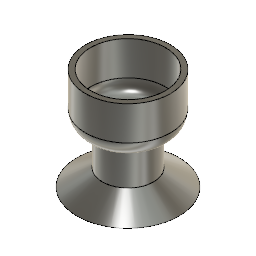
goblet v4 (Autodesk Fusion 360 design; units mm, degrees)
Autodesk Fusion 360 part; units mm, degrees
sketch "outline" plane through (0, 0, 0) normal (0, 1, 0) x (1, 0, 0)
  line L0 (25, -60) -> (25, -40)
  arc A0 (25, -40) -> (15, -30) centre (15, -40) ccw
  line L1 (15, -30) -> (15, -10)
  line L2 (15, -10) -> (30, 0)
  line L3 (30, 0) -> (10, 0)
  line L4 (22, -60) -> (22, -40)
  arc A1 (22, -40) -> (12, -33.6754) centre (15, -40) ccw
  line L5 (12, -33.6754) -> (12, -8.3944)
  line L6 (12, -8.3944) -> (20.0917, -3)
  line L7 (20.0917, -3) -> (10, -3)
  line L8 (22, -60) -> (25, -60)
  line L9 (10, -3) -> (10, 0)
  line L10 (0, -60) -> (0, 0) construction
  dimension "d1" = -3
  dimension "d2" = 20
  dimension "d3" = 10
  dimension "d4" = 20
  dimension "d5" = 18.0278
  dimension "d6" = 20
  constraint vertical L0
  constraint tangent L0 A0
  constraint parallel L0 L1
  constraint horizontal L3
  constraint perpendicular L0 L8
  constraint perpendicular L3 L9
  constraint coincident L10.end origin
  constraint vertical L10
  measures "d2" distance of L0.start L0.end
  measures "d3" radius of A0
  measures "d4" distance of A0.end L1.end
  measures "d5" distance of L1.end L2.end
  measures "d6" distance of L2.end L3.end
revolve "Revolve1" add sketch "outline" angle 360 about axis through (0, 0, 60) along (0, 0, -1)
sketch "Sketch2" plane through (0, 0, 0) normal (0, 0, 1) x (1, 0, 0)
  circle A0 centre (0, 0) radius 10
  constraint coincident A0.centre origin
extrude "Extrude1" add sketch "Sketch2" along normal blind 5
